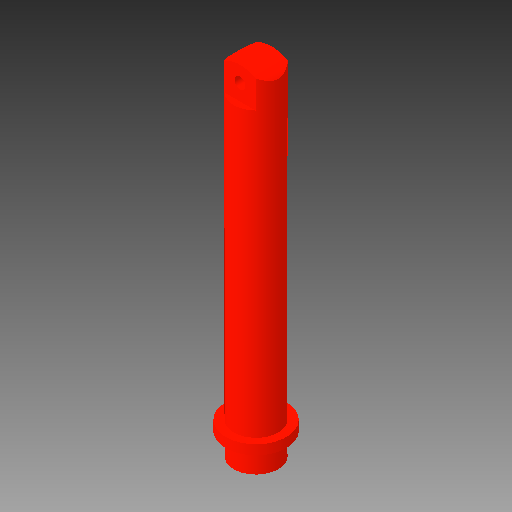
# Autodesk Inventor part: 筷子套
Saved by Autodesk Inventor 2017 (Build 210142000, 142)
## iProperties
Created: 2019-12-02
Part Number: 筷子套
Material: 一般
Document SubType Name: Modeling
Designer: 吳昇峻
Density: 1 g/cm^3
Appearance: 預設
Mass: 13.6217 g
Surface Area: 73.8981 cm^2
Volume: 13.6217 cm^3
Author: 吳昇峻
Autodesk Inventor part; units mm, degrees
ref_plane "YZ Plane" through (0, 0, 0) normal (1, 0, 0) x (0, 1, 0)
ref_plane "XY Plane" through (0, 0, 0) normal (0, 0, 1) x (1, 0, 0)
sketch "草圖1" plane through (0, 0, 0) normal (0, 1, 0) x (-1, 0, 0)
  circle A0 centre (0, 0) radius 3.15
  circle A1 centre (0, 0) radius 7
  dimension "d0" = 6.3
  dimension "d1" = 14
  constraints: 2 centre point, 2 coincident
  measures "d0" diameter of A0
  measures "d1" diameter of A1
extrude "擠出1" add sketch "草圖1" along normal blind 100
sketch "草圖2" plane through (0, 100, 0) normal (0, 1, 0) x (1, 0, 0)
  line L0 (0, 0) -> (0, -5) construction
  circle A0 centre (0, 0) radius 7 projected
  line L1 (-4.899, -5) -> (4.899, -5)
  line L2 (0, 0) -> (0, 5) construction
  line L3 (4.899, 5) -> (-4.899, 5)
  point P0 (-5.3619, -4.5)
  point P1 (-5.3619, 4.5)
  point P2 (5.3619, 4.5)
  dimension "d4" = 5
  dimension "d38" = 5
  constraints: 8 end point, 2 horizontal, 2 vertical, 8 other
  measures "d4" distance of L0.start L0.end
  measures "d38" distance of L2.start L2.end
ref_plane "工作平面1" through (0, 50, 0) normal (0, 1, 0) x (-1, 0, 0)
ref_plane "工作平面2" through (0, 11, 0) normal (0, 1, 0) x (-1, 0, 0)
sketch "草圖10" plane through (0, 11, 0) normal (0, 1, 0) x (-1, 0, 0)
  circle A0 centre (0, 0) radius 3.15
  circle A1 centre (0, 0) radius 9.5
  dimension "d30" = 6.3
  dimension "d31" = 19
  constraints: 2 centre point, 2 coincident
  measures "d30" diameter of A0
  measures "d31" diameter of A1
extrude "擠出9" add sketch "草圖10" against normal blind 3
extrude "擠出11" add sketch "草圖2" along normal blind 10 contours A0 L1 L3
sketch "草圖12" plane through (4.899, 100, -5) normal (0, 0, -1) x (-1, 0, 0)
  circle A0 centre (4.899, 5) radius 1.75
  line L0 (9.798, 0) -> (0, 0) projected
  arc A1 (11.899, 7.1414) -> (-2.101, 7.1414) centre (4.899, 0) ccw
  line L1 (-2.101, -89) -> (-2.101, 10) projected
  line L2 (-2.101, 7.1414) -> (-2.101, 0)
  line L3 (-2.101, -89) -> (-2.101, 10) projected
  line L4 (11.899, -89) -> (11.899, 10) projected
  line L5 (11.899, 0) -> (-2.101, 0)
  line L6 (11.899, -89) -> (11.899, 10) projected
  line L7 (11.899, 0) -> (11.899, 7.1414)
  line L8 (11.899, -89) -> (11.899, 10) projected
  line L9 (-2.101, 7.1414) -> (-2.101, 10)
  line L10 (0, 10) -> (-2.101, 10) projected
  line L11 (11.899, 10) -> (-2.101, 10)
  line L12 (11.899, 7.1414) -> (11.899, 10)
  point P0 (4.899, -100)
  dimension "d41" = 3.5
  dimension "d44" = 20
  constraints: 12 end point, 5 point on line, 2 centre point, 2 collinear, 2 point on circle, 1 horizontal, 1 midpoint, 1 perpendicular
  measures "d41" diameter of A0
  measures "d44" diameter of A1
extrude "擠出12" cut sketch "草圖12" against normal up to next contours A0
extrude "擠出13" cut sketch "草圖12" against normal up to next contours A1 L11 L4 | L1 L10 L11 A1
sketch "Sketch13" plane through (0, 0, 0) normal (0, -1, 0) x (1, 0, 0)
  circle A0 centre (0, 0) radius 7 projected
  circle A1 centre (0, 0) radius 7
  constraints: 1 centre point, 1 coincident
extrude "Extrusion14" cut sketch "Sketch13" against normal blind 1
